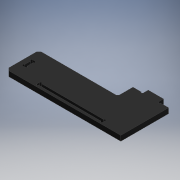
# Autodesk Inventor part: コックピット_2_メインフレーム_2
Saved by Autodesk Inventor 2018 (Build 220112000, 112)
## iProperties
Created: 2016-05-24
Part Number: コックピット_2_メインフレーム_2
Material: アセタール樹脂、黒
Document SubType Name: Modeling
Designer: hiroaki
Density: 1.425 g/cm^3
Appearance: 滑らか - 黒
Mass: 17.4619 g
Surface Area: 93.6545 cm^2
Volume: 12.254 cm^3
Author: hiroaki
Autodesk Inventor part; units mm, degrees
ref_plane "YZ Plane" through (0, 0, 0) normal (1, 0, 0) x (0, 1, 0)
ref_plane "XZ Plane" through (0, 0, 0) normal (0, 1, 0) x (-1, 0, 0)
ref_plane "XY Plane" through (0, 0, 0) normal (0, 0, 1) x (1, 0, 0)
derived "コックピット_2_基礎_2.ipt"
sketch "スケッチ1" plane through (0, 0, 0) normal (0, 0, 1) x (1, 0, 0)
  line L0 (-55, 16) -> (-55, -16) construction
  line L1 (-55, -16) -> (55, -16)
  line L2 (55, -16) -> (55, 31)
  line L3 (55, 31) -> (47.1, 31)
  line L4 (-55, 16) -> (20, 16)
  line L5 (20, 16) -> (20, 31)
  line L6 (20, 31) -> (27.9, 31)
  line L7 (30, 31) -> (30, 36)
  line L8 (30, 36) -> (45, 36)
  line L9 (45, 36) -> (45, 31)
  arc A0 (27.9, 31) -> (30, 31) centre (28.95, 31) ccw
  arc A1 (45, 31) -> (47.1, 31) centre (46.05, 31) ccw
  line L10 (37.5, 36) -> (37.5, -16) construction
  line L11 (-55, 16) -> (-50, 16) construction
  line L12 (-50, 16) -> (-50, -16) construction
  line L13 (-50, -16) -> (-55, -16) construction
  line L14 (-55, -16) -> (-55, 16) construction
  line L15 (-50, -16) -> (55, -16) construction
  line L16 (55, -16) -> (55, -11) construction
  line L17 (55, -11) -> (-50, -11) construction
  line L18 (-50, -11) -> (-50, -16) construction
  circle A2 centre (-52.5, 12) radius 1.55
  circle A3 centre (-52.5, -12) radius 1.55
  line L19 (-55, 0) -> (-50, 0) construction
  line L20 (-55, 16) -> (-57.5, 13.5)
  line L21 (-57.5, 13.5) -> (-57.5, -13.5)
  line L22 (-57.5, -13.5) -> (-55, -16)
  circle A4 centre (-52.5, 12) radius 3 construction
  line L23 (-50, 5) -> (-52.5, 5) construction
  line L24 (-52.5, 5) -> (-52.5, -5) construction
  line L25 (-52.5, -5) -> (-50, -5) construction
  line L26 (-50, -5) -> (-50, 5) construction
  line L27 (-30, -11) -> (35, -11) construction
  line L28 (35, -11) -> (35, -13.5) construction
  line L29 (35, -13.5) -> (-30, -13.5) construction
  line L30 (-30, -13.5) -> (-30, -11) construction
  line L31 (-52.55, -5.05) -> (-52.55, 5.05)
  line L32 (-52.55, 5.05) -> (-49.95, 5.05)
  line L33 (-49.95, 5.05) -> (-49.95, -5.05)
  line L34 (-49.95, -5.05) -> (-52.55, -5.05)
  circle A5 centre (-52.55, -4) radius 1.05
  circle A6 centre (-49.95, -4) radius 1.05
  circle A7 centre (-52.55, 4) radius 1.05
  circle A8 centre (-49.95, 4) radius 1.05
  line L35 (-30.05, -10.95) -> (35.05, -10.95)
  line L36 (35.05, -10.95) -> (35.05, -13.55)
  line L37 (35.05, -13.55) -> (-30.05, -13.55)
  line L38 (-30.05, -13.55) -> (-30.05, -10.95)
  circle A9 centre (-29, -13.55) radius 1.05
  circle A10 centre (-29, -10.95) radius 1.05
  circle A11 centre (34, -10.95) radius 1.05
  circle A12 centre (34, -13.55) radius 1.05
  point P0 (0, 0)
  point P1 (0, -16)
  point P2 (-52.5, 16)
  dimension "d13" = 2.1
  dimension "d14" = 0.05
  dimension "d15" = 0.05
  measures "d14" distance between parallel lines of L31 L24
  measures "d15" distance between parallel lines of L38 L30
extrude "押し出し1" add sketch "スケッチ1" along normal blind 5
fillet "フィレット1" radius 2 1 edges at (20, 16, 2.5)
sketch "スケッチ6" plane through (55, -16, 0) normal (0, 0, -1) x (-1, 0, 0)
  circle A0 centre (107.5, 28) radius 1.55 projected
  circle A1 centre (107.5, 28) radius 1.55
  circle A2 centre (107.5, 4) radius 1.55 projected
  circle A3 centre (107.5, 4) radius 1.55
  point P0 (55, 16)
  constraints: 2 centre point, 2 coincident
extrude "押し出し3" add sketch "スケッチ6" against normal up to surface (5 mm away)
